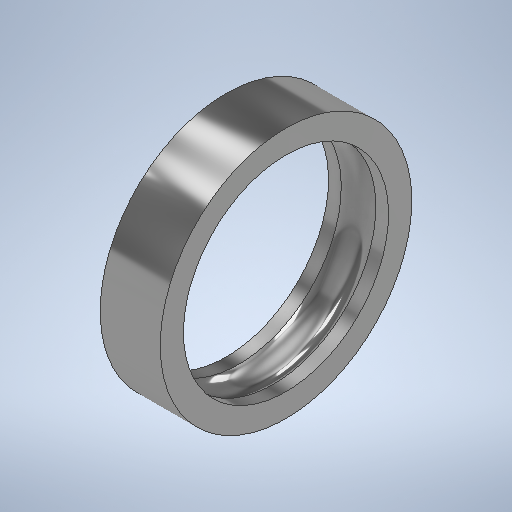
# Autodesk Inventor part: Outer ring
Saved by Autodesk Inventor 2025.1 (Build 291241000, 241)
## iProperties
Created: 2024-08-09
Part Number: Outer ring
Material: Generic
Document SubType Name: Modeling
Designer: vedan
Density: 1 g/cm^3
Appearance: Chrome - Polished Black
Author: vedan
Autodesk Inventor part; units mm, degrees
ref_plane "XY Plane" through (0, 0, 0) normal (0, 0, 1) x (1, 0, 0)
sketch "Sketch1" plane through (0, 0, 0) normal (0, 0, 1) x (1, 0, 0)
  line L0 (15.5, 53) -> (15.5, 65)
  line L1 (15.5, 65) -> (-15.5, 65)
  line L2 (-15.5, 65) -> (-15.5, 53)
  line L3 (-15.5, 53) -> (15.5, 65) construction
  line L4 (15.5, 53) -> (-15.5, 65) construction
  line L5 (0, 53) -> (0, 45) construction
  arc A0 (8.9443, 53) -> (-8.9443, 53) centre (0, 45) ccw
  line L6 (-15.5, 53) -> (-8.9443, 53)
  line L7 (8.9443, 53) -> (15.5, 53)
  line L8 (-8.9443, 53) -> (8.9443, 53) construction
  line L9 (-16.6622, 0) -> (29.8943, 0) construction
  line L10 (0, 45) -> (0, 0) construction
  point P0 (0, 57)
  dimension "d1" = 31
  dimension "d2" = 12
  dimension "d3" = 53
  dimension "d4" = 8
  dimension "d6" = 12
  constraints: 22 end point, 4 horizontal, 3 parallel, 3 point on circle, 2 perpendicular, 2 vertical, 1 centre point, 1 coincident
  measures "d1" distance of L1.end L0.end
  measures "d2" distance of L0.end L0.start
  measures "d3" distance of L10.end L5.start
  measures "d4" distance of L5.start L5.end
  measures "d6" distance of point (0, 57) L5.end
revolve "Revolution1" add sketch "Sketch1" angle 360 about axis through (-16.6622, 0, 0) along (1, 0, 0)
ref_plane "Work Plane1" through (0, 0, 0) normal (1, 0, 0) x (0, 1, 0)
body "Solid1"
